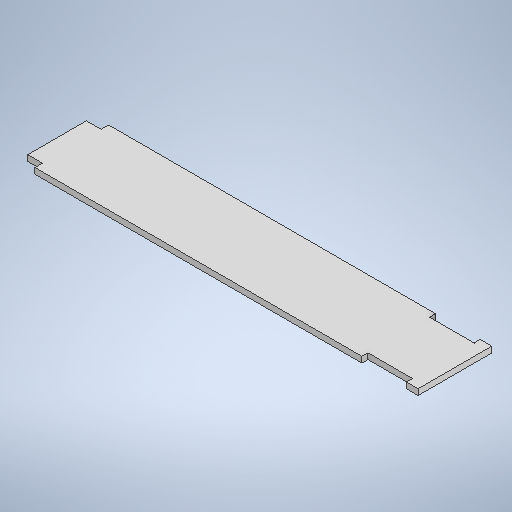
# Autodesk Inventor part: 우측 센서 막대기
Saved by Autodesk Inventor 2025 (Build 290162000, 162)
## iProperties
Created: 2024-05-11
Part Number: 우측 센서 막대기
Material: 일반
Document SubType Name: Modeling
Designer: gmsee
Density: 1 g/cm^3
Appearance: 기본값
Author: gmsee
Autodesk Inventor part; units mm, degrees
ref_plane "YZ Plane" through (0, 0, 0) normal (1, 0, 0) x (0, 1, 0)
ref_plane "XZ Plane" through (0, 0, 0) normal (0, 1, 0) x (-1, 0, 0)
ref_plane "XY Plane" through (0, 0, 0) normal (0, 0, 1) x (1, 0, 0)
sketch "스케치1" plane through (0, 0, 0) normal (0, 1, 0) x (-1, 0, 0)
  line L0 (-199.7433, 25.7945) -> (-199.7433, -24.2055)
  line L1 (-149.7433, 25.7945) -> (-149.7433, -24.2055) construction
  line L2 (-161.6433, 25.7945) -> (-161.6433, 21.6945)
  line L3 (-161.6433, 21.6945) -> (-191.8433, 21.6945)
  line L4 (-191.8433, 21.6945) -> (-191.8433, 25.7945)
  line L5 (-153.7433, 25.7945) -> (-153.7433, -24.2055) construction
  line L6 (-161.6433, -24.2055) -> (-161.6433, -20.1055)
  line L7 (-161.6433, -20.1055) -> (-191.8433, -20.1055)
  line L8 (-191.8433, -20.1055) -> (-191.8433, -24.2055)
  line L9 (60.2567, 25.7945) -> (60.2567, 20.6945)
  line L10 (60.2567, 20.6945) -> (70.2567, 20.6945)
  line L11 (70.2567, 20.6945) -> (70.2567, -19.1055)
  line L12 (70.2567, -19.1055) -> (60.2567, -19.1055)
  line L13 (60.2567, -19.1055) -> (60.2567, -24.2055)
  line L14 (60.2567, -24.2055) -> (-161.6433, -24.2055)
  line L15 (-191.8433, -24.2055) -> (-199.7433, -24.2055)
  line L16 (60.2567, 25.7945) -> (-161.6433, 25.7945)
  line L17 (-191.8433, 25.7945) -> (-199.7433, 25.7945)
  point P0 (0, 0)
  point P1 (-199.7433, 0.7945)
  point P2 (-149.7433, 0.7945)
  point P3 (-161.6433, 23.7445)
  point P4 (-161.6433, -22.1555)
  point P5 (-195.7933, -24.2055)
  dimension "d2" = 260
  dimension "d4" = 50
  dimension "d5" = 4.1
  dimension "d6" = 30.2
  dimension "d7" = 4
  dimension "d8" = 7.9
  dimension "d9" = 4.1
  dimension "d10" = 30.2
  dimension "d11" = 7.9
  dimension "d12" = 5.1
  dimension "d13" = 5.1
  dimension "d14" = 10
  dimension "d17" = 50
  constraints: 36 end point, 14 perpendicular, 5 midpoint, 5 point on line, 4 horizontal, 3 vertical
  measures "d2" distance of L13.end L0.end
  measures "d4" distance of point (-199.743, 0.794) point (-149.743, 0.794)
  measures "d5" distance of L2.start L2.end
  measures "d6" distance of L2.end L4.start
  measures "d7" distance between parallel lines of L1 L5
  measures "d8" distance from line of L5 point (-161.643, 23.744)
  measures "d9" distance of L6.start L6.end
  measures "d10" distance of L6.end L7.end
  measures "d11" distance from line of point (-161.643, -22.156) L5
  measures "d12" distance of L9.start L9.end
  measures "d13" distance of L12.end L13.end
  measures "d14" distance of L11.end L12.end
  measures "d17" distance from line of point (-195.793, -24.206) L17
extrude "돌출1" add sketch "스케치1" along normal blind 4
